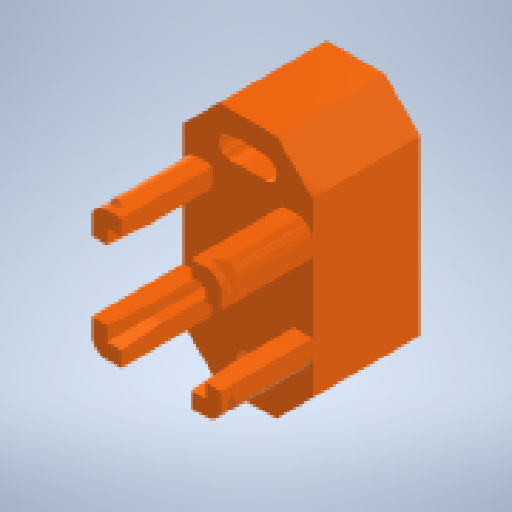
# Autodesk Inventor part: MicroRail-FlextureBase-CubeAttachment
Saved by Autodesk Inventor 2023.1 (Build 271208000, 208)
## iProperties
Created: 2023-06-05
Part Number: MicroRail-FlextureBase-CubeAttachment
Material: ABS Plastic
Document SubType Name: Modeling
Designer: hello
Density: 1.06 g/cm^3
Appearance: Smooth - Light Orange
Author: hello
Autodesk Inventor part; units mm, degrees
ref_plane "YZ Plane" through (0, 0, 0) normal (1, 0, 0) x (0, 1, 0)
ref_plane "XZ Plane" through (0, 0, 0) normal (0, 1, 0) x (-1, 0, 0)
ref_plane "XY Plane" through (0, 0, 0) normal (0, 0, 1) x (1, 0, 0)
sketch "Sketch1" plane through (0, 0, 0) normal (0, 0, 1) x (1, 0, 0)
  line L0 (-9, -17) -> (9, -17)
  line L1 (9, -17) -> (9, 17)
  line L2 (9, 17) -> (-9, 17)
  line L3 (-9, 17) -> (-9, -17)
  line L4 (-9, -17) -> (9, 17) construction
  line L5 (9, -17) -> (-9, 17) construction
  line L6 (0, -12.5) -> (0, 12.5) construction
  circle A0 centre (0, -12.5) radius 1.55
  arc A1 (2.5, 12.3747) -> (-2.5, 12.3747) centre (0, -12.5) ccw construction
  arc A2 (2.652, 13.8871) -> (-2.652, 13.8871) centre (0, -12.5) ccw
  arc A3 (2.348, 10.8623) -> (-2.348, 10.8623) centre (0, -12.5) ccw
  arc A4 (2.348, 10.8623) -> (2.652, 13.8871) centre (2.5, 12.3747) ccw
  arc A5 (-2.652, 13.8871) -> (-2.348, 10.8623) centre (-2.5, 12.3747) ccw
  point P0 (0, 0)
  dimension "d0" = 18
  dimension "d1" = 34
  dimension "d4" = 25
  dimension "d5" = 3.1
  dimension "d18" = 1.52
  dimension "d20" = 5
  constraints: 14 end point, 11 point on circle, 6 centre point, 4 tangent, 3 midpoint, 2 parallel, 1 coincident, 1 horizontal, 1 horizontal alignment, 1 perpendicular, 1 vertical, 1 vertical alignment
  measures "d0" distance of L2.end L1.end
  measures "d1" distance of L1.end L0.end
  measures "d4" distance of L6.end L6.start
  measures "d5" diameter of A0
  measures "d18" radius of A4
  measures "d20" distance of A1.end A1.start
extrude "Extrusion1" add sketch "Sketch1" along normal blind 15
chamfer "Chamfer1" distance 5 angle 45 4 edges at (9, -17, 7.5) (-9, -17, 7.5) (-9, 17, 7.5) (9, 17, 7.5)
sketch "Sketch3" plane through (0, 0, 15) normal (0, 0, 1) x (1, 0, 0)
  line L0 (6.35, -6.35) -> (-6.35, -6.35)
  line L1 (-6.35, -6.35) -> (-6.35, 6.35)
  line L2 (-6.35, 6.35) -> (6.35, 6.35)
  line L3 (6.35, 6.35) -> (6.35, -6.35)
  line L4 (6.35, -6.35) -> (-6.35, 6.35) construction
  line L5 (-6.35, -6.35) -> (6.35, 6.35) construction
  line L6 (9, -12) -> (9, 12) projected
  line L7 (-9, -9) -> (9, -9)
  line L8 (9, -9) -> (9, 9)
  line L9 (9, 9) -> (-9, 9)
  line L10 (-9, 9) -> (-9, -9)
  line L11 (9, -4.85) -> (-9, -4.85)
  line L12 (9, 4.85) -> (7.7149, 4.85)
  line L13 (7.7149, 4.85) -> (-9, 4.85)
  line L14 (-9, 12) -> (-9, -12) projected
  line L15 (4.85, -9) -> (4.85, 9)
  line L16 (-4.85, -9) -> (-4.85, 9)
  point P0 (0, 0)
  point P1 (-4.85, -6.35)
  point P2 (-6.35, -4.85)
  point P3 (-4.85, 6.35)
  point P4 (-6.35, 4.85)
  point P5 (4.85, 6.35)
  point P6 (6.35, 4.85)
  point P7 (4.85, -6.35)
  point P8 (6.35, -4.85)
  dimension "d11" = 12.7
  dimension "d12" = 1.5
  dimension "d13" = 1.5
  dimension "d14" = 1.5
  dimension "d15" = 1.5
  constraints: 30 end point, 10 point on line, 7 perpendicular, 4 parallel, 2 midpoint, 1 horizontal, 3 other
  measures "d11" distance of L1.end L2.end
  measures "d12" distance from line of L1.end L16
  measures "d13" distance between parallel lines of L15 L3
  measures "d14" distance from line of L11 L0.start
  measures "d15" distance from line of L2.end L13
extrude "Extrusion2" add sketch "Sketch3" along normal blind 12.7 contours L3 L11 L6 L7 L15 L0 | L16 L7 L10 L11 L1 L0 | L3 L2 L15 L9 L6 L12 L13 | L13 L10 L9 L16 L2 L1
fillet "Fillet1" radius 2 4 edges at (9, -9, 21.35) (9, 9, 21.35) (-9, 9, 21.35) (-9, -9, 21.35)
sketch "Sketch4" plane through (0, 0, 0) normal (1, 0, 0) x (0, 1, 0)
  line L0 (11, 26.7) -> (13, 26.7)
  line L1 (13, 26.7) -> (13, 24.1)
  line L2 (13, 24.1) -> (11, 26.1)
  line L3 (11, 26.1) -> (11, 26.7)
  line L4 (0, 0) -> (0, 19.6238)
  line L5 (7, 27.7) -> (9, 27.7) projected
  dimension "d22" = 0.6
  dimension "d23" = 22
  dimension "d24" = 1
  dimension "d25" = 135
  dimension "d26" = 2
  constraints: 10 end point, 1 horizontal, 1 parallel, 1 perpendicular, 1 vertical
  measures "d22" distance of L2.end L0.start
  measures "d23" diameter of L3 L4
  measures "d24" distance between parallel lines of L5 L0
  measures "d25" angle of L2 L3
  measures "d26" distance of L0.start L0.end
revolve "Revolution1" cut sketch "Sketch4" angle 360 about axis through (0, 0, 0) along (0, 0, 1)
chamfer "Chamfer2" distance 0.5 angle 85 2 edges at (5.6, -6.35, 27.7) (6.35, -5.6, 27.7) measured on face at (5.6, -6.85, 27.7) measured on face at (6.85, -5.6, 27.7)
chamfer "Chamfer3" distance 0.5 angle 85 2 edges at (6.35, 5.6, 27.7) (5.6, 6.35, 27.7) measured on face at (6.85, 5.6, 27.7) measured on face at (5.6, 6.85, 27.7)
chamfer "Chamfer4" distance 0.5 angle 85 2 edges at (-5.6, 6.35, 27.7) (-6.35, 5.6, 27.7) measured on face at (-5.6, 6.85, 27.7) measured on face at (-6.85, 5.6, 27.7)
chamfer "Chamfer5" distance 0.5 angle 85 2 edges at (-5.6, -6.35, 27.7) (-6.35, -5.6, 27.7) measured on face at (-6.85, -5.6, 27.7) measured on face at (-5.6, -6.85, 27.7)
body "Solid1"
